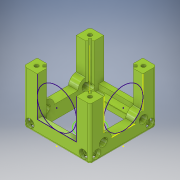
# Autodesk Inventor part: 10_Cube_v0_B
Saved by Autodesk Inventor 2019 (Build 230136000, 136)
## iProperties
Created: 2018-05-19
Part Number: 10_Cube_v0_B
Material: Generisch
Document SubType Name: Modeling
Designer: diederichbenedict
Density: 1 g/cm^3
Appearance: IPHT_Grün
Mass: 20.3218 g
Surface Area: 129.075 cm^2
Volume: 20.3218 cm^3
Author: diederichbenedict
Autodesk Inventor part; units mm, degrees
ref_plane "YZ Plane" through (0, 0, 0) normal (1, 0, 0) x (0, 1, 0)
ref_plane "XZ Plane" through (0, 0, 0) normal (0, 1, 0) x (-1, 0, 0)
sketch "Skizze1" plane through (0, 0, 0) normal (0, 0, 1) x (1, 0, 0)
  line L0 (-24.9, 24.9) -> (24.9, 24.9)
  line L1 (24.9, 24.9) -> (24.9, -24.9)
  line L2 (24.9, -24.9) -> (-24.9, -24.9)
  line L3 (-24.9, -24.9) -> (-24.9, 24.9)
  line L4 (-24.9, 24.9) -> (24.9, -24.9) construction
  line L5 (24.9, 24.9) -> (-24.9, -24.9) construction
  line L6 (14.6269, -17.9) -> (-14.6269, -17.9)
  line L7 (-17.9, -14.6269) -> (-17.9, 14.6269)
  line L8 (-14.6269, 17.9) -> (14.6269, 17.9)
  line L9 (17.9, 14.6269) -> (17.9, -14.6269)
  line L10 (20.5, -20.5) -> (-20.5, 20.5) construction
  line L11 (-20.5, -20.5) -> (20.5, 20.5) construction
  line L12 (-14.6269, 17.9) -> (-17.9, 14.6269)
  line L13 (-14.6269, 17.9) -> (-9.9981, 17.9) construction
  line L14 (17.9, -14.6269) -> (14.6269, -17.9)
  line L15 (17.9, -14.6269) -> (22.5288, -14.6269) construction
  line L16 (-17.9, -14.6269) -> (-14.6269, -17.9)
  line L17 (14.6269, 17.9) -> (17.9, 14.6269)
  point P0 (0, 0)
  dimension "d0" = 49.8
  dimension "d1" = 49.8
  dimension "d2" = 41
  dimension "d3" = 41
  dimension "d4" = 135
  dimension "d5" = 23
  dimension "d6" = 135
  dimension "d7" = 23
  dimension "a1" = 23
  dimension "d9" = 23
  dimension "a2" = 7
  dimension "d42" = 7
  dimension "d43" = 7
  dimension "d44" = 7
  constraints: 36 end point, 4 horizontal, 4 midpoint, 4 parallel, 4 perpendicular, 2 equal length
  measures "d0" distance of L1.end L2.end
  measures "d1" distance of L0.end L1.end
  measures "d2" distance of L10.end L11.end
  measures "d3" distance of L11.start L10.end
  measures "d4" angle of L12 L13
  measures "d5" distance from line of point (0, 0) L12
  measures "d6" angle of L14 L15
  measures "d7" distance from line of point (0, 0) L14
  measures "a1" distance from line of point (0, 0) L17
  measures "d9" distance from line of L16 point (0, 0)
  measures "a2" distance between parallel lines of L8 L0
  measures "d42" distance between parallel lines of L3 L7
  measures "d43" distance between parallel lines of L2 L6
  measures "d44" distance between parallel lines of L1 L9
extrude "Extrusion1" add sketch "Skizze1" along normal blind 10.3
sketch "Skizze2" plane through (0, 0, 10.3) normal (0, 0, 1) x (1, 0, 0)
  line L0 (-17.9, 14.6269) -> (-14.6269, 17.9) construction
  line L1 (-14.6269, 17.9) -> (14.6269, 17.9) construction
  line L2 (14.6269, 17.9) -> (17.9, 14.6269) construction
  line L3 (17.9, 14.6269) -> (17.9, -14.6269) construction
  line L4 (17.9, -14.6269) -> (14.6269, -17.9) construction
  line L5 (14.6269, -17.9) -> (-14.6269, -17.9) construction
  line L6 (-14.6269, -17.9) -> (-17.9, -14.6269) construction
  line L7 (-17.9, -14.6269) -> (-17.9, 14.6269) construction
  line L8 (24.9, 24.9) -> (-24.9, 24.9) construction
  line L9 (-24.9, 24.9) -> (-24.9, -24.9) construction
  line L10 (-24.9, -24.9) -> (24.9, -24.9) construction
  line L11 (24.9, -24.9) -> (24.9, 24.9) construction
  line L12 (-17.9, -14.6269) -> (-24.9, -14.6269)
  line L13 (-24.9, -24.9) -> (-24.9, 24.9) projected
  line L14 (-24.9, -14.6269) -> (-24.9, -24.9)
  line L15 (-17.9, -14.6269) -> (-14.6269, -17.9) projected
  line L16 (-17.9, -14.6269) -> (-14.6269, -17.9)
  line L17 (-14.6269, -17.9) -> (-14.6269, -24.9)
  line L18 (24.9, -24.9) -> (-24.9, -24.9) projected
  line L19 (-24.9, -24.9) -> (-14.6269, -24.9)
  line L20 (-17.9, -14.9) -> (-17.9, 14.9) projected
  line L21 (14.9, -17.9) -> (-14.9, -17.9) projected
  line L22 (17.9, 14.9) -> (17.9, -14.9) projected
  line L23 (-14.9, 17.9) -> (-9.9, 17.9) projected
  circle A0 centre (0, 0) radius 17.9
  line L24 (14.6269, -17.9) -> (17.9, -14.6269)
  line L25 (17.9, -14.6269) -> (24.9, -14.6269)
  line L26 (24.9, -24.9) -> (24.9, -14.6269)
  line L27 (14.6269, -24.9) -> (24.9, -24.9)
  line L28 (14.6269, -17.9) -> (14.6269, -24.9)
  line L29 (17.9, 14.6269) -> (14.6269, 17.9)
  line L30 (14.6269, 17.9) -> (14.6269, 24.9)
  line L31 (24.9, 24.9) -> (14.6269, 24.9)
  line L32 (24.9, 14.6269) -> (24.9, 24.9)
  line L33 (17.9, 14.6269) -> (24.9, 14.6269)
  line L34 (-14.6269, 17.9) -> (-17.9, 14.6269)
  line L35 (-17.9, 14.6269) -> (-24.9, 14.6269)
  line L36 (-24.9, 24.9) -> (-24.9, 14.6269)
  line L37 (-14.6269, 24.9) -> (-24.9, 24.9)
  line L38 (-14.6269, 17.9) -> (-14.6269, 24.9)
  line L39 (0, 0) -> (24.9, -24.9) construction
  line L40 (14.4957, -15.9099) -> (16.617, -18.0312)
  line L41 (16.617, -18.0312) -> (18.0312, -16.617)
  line L42 (18.0312, -16.617) -> (15.9099, -14.4957)
  line L43 (15.9099, -14.4957) -> (14.4957, -15.9099)
  line L44 (14.4957, -15.9099) -> (18.0312, -16.617) construction
  line L45 (16.617, -18.0312) -> (15.9099, -14.4957) construction
  line L46 (14.6269, -17.9) -> (17.9, -14.6269) projected
  point P0 (16.2635, -16.2635)
  point P1 (16.9706, -15.5563)
  point P2 (15.5563, -16.9706)
  dimension "d80" = 360
  dimension "d101" = 3
  dimension "d102" = 2
  constraints: 54 end point, 6 point on line, 5 midpoint, 3 perpendicular, 3 tangent, 2 collinear, 2 parallel, 1 centre point, 1 vertical, 41 other
  measures "d101" distance of L40.start L40.end
  measures "d102" distance of L41.end L40.end
extrude "Extrusion2" add sketch "Skizze2" along normal blind 29.4 contours L15 L17 L18 L13 L12 | L29 L30 L31 L32 L33 | L13 L37 L38 L34 L35 | L28 L24 L40 L41 L42 L25 L26 L18 | L24 L42 L41 L40
fillet "Rundung1" radius 2 8 edges at (24.9, 24.9, 19.85) (24.9, 0, 0) (24.9, -24.9, 19.85) (-24.9, 24.9, 19.85) (-24.9, -24.9, 19.85) (-24.9, 0, 0) (0, -24.9, 0) (0, 24.9, 0)
sketch "Skizze3" plane through (0, 0, 39.7) normal (0, 0, 1) x (1, 0, 0)
  line L0 (20, 20) -> (-20, 20) construction
  line L1 (-20, 20) -> (-20, -20) construction
  line L2 (-20, -20) -> (20, -20) construction
  line L3 (20, -20) -> (20, 20) construction
  line L4 (20, 20) -> (-20, -20) construction
  line L5 (-20, 20) -> (20, -20) construction
  line L6 (22.9, -22.9) -> (20.7681, -22.9) projected
  line L7 (22.9, -20.7681) -> (22.9, -22.9) projected
  arc A0 (20.7681, -22.9) -> (22.9, -20.7681) centre (20, -20) ccw projected
  point P0 (0, 0)
  point P1 (-20, 20)
  point P2 (20, -20)
  point P3 (20, -20)
  point P4 (20, -20)
  point P5 (-20, -20)
  point P6 (-20, -20)
  point P7 (-15.7881, 5.2)
  point P8 (-15.7881, -5.2)
  dimension "d15" = 40
  dimension "d16" = 40
  constraints: 12 end point, 2 midpoint, 2 parallel, 1 horizontal, 1 perpendicular
  measures "d15" distance of L2.end L1.end
  measures "d16" distance of L1.end L0.end
hole "Bohrung1" at (20, -20, 39.7) at (-20, -20, 39.7) at (-20, 20, 39.7) at (20, 20, 39.7) direction (0, 0, -1) diameter 2.9 depth 10 tip angle 118
sketch "Skizze4" plane through (0, 0, 0) normal (0, 0, -1) x (-1, 0, 0)
  circle A0 centre (20, -20) radius 1.45 projected
  circle A1 centre (20, 20) radius 1.45 projected
  line L0 (14.6269, 17.9) -> (17.9, 14.6269) projected
  line L1 (17.9, 14.6269) -> (17.9, -14.6269) projected
  line L2 (17.9, -14.6269) -> (14.6269, -17.9) projected
  line L3 (14.6269, -17.9) -> (-14.6269, -17.9) projected
  line L4 (-14.6269, -17.9) -> (-17.9, -14.6269) projected
  line L5 (-17.9, -14.6269) -> (-17.9, 14.6269) projected
  line L6 (-17.9, 14.6269) -> (-14.6269, 17.9) projected
  line L7 (-14.6269, 17.9) -> (14.6269, 17.9) projected
  line L8 (-22.9, 22.9) -> (22.9, 22.9) projected
  line L9 (-22.9, -22.9) -> (-22.9, 22.9) projected
  line L10 (22.9, -22.9) -> (-22.9, -22.9) projected
  line L11 (22.9, 22.9) -> (22.9, -22.9) projected
  circle A2 centre (-20, -20) radius 1.45 projected
  circle A3 centre (-20, 20) radius 1.45 projected
  point P0 (0, 0)
  point P1 (19.8136, -18.5116)
  point P2 (18.5116, -19.8136)
  point P3 (18.5116, 19.8136)
  point P4 (19.8136, 18.5116)
  point P5 (-18.5116, -19.8136)
  point P6 (-19.8136, -18.5116)
  point P7 (-19.8136, 18.5116)
  point P8 (-18.5116, 19.8136)
  constraints: 6 other
hole "Bohrung2" at (-20, -20, 0) at (-20, 20, 0) at (20, -20, 0) at (20, 20, 0) direction (0, 0, 1) diameter 3 depth 15 tip angle 118 counterbore diameter 6.2 counterbore depth 2.5
sketch "Skizze8" plane through (24.9, -14.6269, 10.3) normal (1, 0, 0) x (0, 0, -1)
  line L0 (-39.7, 33.8588) -> (-39.7, -4.605) projected
  arc A0 (-37.7, 39.5269) -> (-39.7, 37.5269) centre (-37.7, 37.5269) ccw projected
  arc A1 (8.3, -10.2731) -> (10.3, -8.2731) centre (8.3, -8.2731) ccw projected
  arc A2 (-39.7, -8.2731) -> (-37.7, -10.2731) centre (-37.7, -8.2731) ccw projected
  arc A3 (10.3, 37.5269) -> (8.3, 39.5269) centre (8.3, 37.5269) ccw projected
  line L1 (-37.7, -8.2731) -> (8.3, 37.5269) construction
  line L2 (8.3, -8.2731) -> (8.3, 37.5269) construction
  line L3 (8.3, -8.2731) -> (-37.7, 37.5269) construction
  circle A4 centre (-14.7, 14.6269) radius 6.587 construction
  line L4 (-34.7, -5.3731) -> (5.3, -5.3731) construction
  line L5 (5.3, -5.3731) -> (5.3, 34.6269) construction
  line L6 (5.3, 34.6269) -> (-34.7, 34.6269) construction
  line L7 (-34.7, 34.6269) -> (-34.7, -5.3731) construction
  line L8 (-34.7, -5.3731) -> (5.3, 34.6269) construction
  line L9 (5.3, -5.3731) -> (-34.7, 34.6269) construction
  point P0 (10.3, 14.6269)
  dimension "d110" = 40
  dimension "d111" = 40
  constraints: 16 end point, 3 midpoint, 2 parallel, 1 centre point, 1 horizontal, 1 perpendicular
  measures "d110" distance of L6.end L5.end
  measures "d111" distance of L5.end L4.end
sketch "Skizze9" plane through (14.6269, 17.9, 10.3) normal (-1, 0, 0) x (0, 0, 1)
  line L0 (-3.2288, -37.966) -> (32.6288, -37.966) construction
  line L1 (32.6288, -37.966) -> (34.766, -35.8288) construction
  line L2 (34.766, -35.8288) -> (34.766, 0.0288) construction
  line L3 (34.766, 0.0288) -> (32.6288, 2.166) construction
  line L4 (32.6288, 2.166) -> (-3.2288, 2.166) construction
  line L5 (-3.2288, 2.166) -> (-5.366, 0.0288) construction
  line L6 (-5.366, 0.0288) -> (-5.366, -35.8288) construction
  line L7 (-5.366, -35.8288) -> (-3.2288, -37.966) construction
  circle A0 centre (29.7, -2.9) radius 3.2639 construction
  circle A1 centre (-0.3, -2.9) radius 3.2639 construction
  circle A2 centre (-0.3, -32.9) radius 3.2639 construction
  circle A3 centre (29.7, -32.9) radius 3.2639 construction
  circle A4 centre (14.7, -17.9) radius 13.3985 construction
  line L8 (-3.643, 3.166) -> (33.043, 3.166)
  line L9 (33.043, 3.166) -> (35.766, 0.443)
  line L10 (35.766, 0.443) -> (35.766, -36.243)
  line L11 (35.766, -36.243) -> (33.043, -38.966)
  line L12 (33.043, -38.966) -> (-3.643, -38.966)
  line L13 (-3.643, -38.966) -> (-6.366, -36.243)
  line L14 (-6.366, -36.243) -> (-6.366, 0.443)
  line L15 (-6.366, 0.443) -> (-3.643, 3.166)
  point P0 (-10.3, -17.9)
  dimension "d82" = 1
  constraints: 16 end point, 7 other
  measures "d82" distance between parallel lines of L4 L8
extrude "Extrusion5" cut sketch "Skizze9" along normal up to surface (29.2538 mm away)
sketch "Skizze10" plane through (-24.9, -14.6269, 10.3) normal (-1, 0, 0) x (0, 0, 1)
  circle A0 centre (-0.3, 29.6269) radius 3.2639 construction
  circle A1 centre (-0.3, -0.3731) radius 3.2639 construction
  circle A2 centre (29.7, 29.6269) radius 3.2639 construction
  circle A3 centre (29.7, -0.3731) radius 3.2639 construction
  circle A4 centre (29.7, 29.6269) radius 3.3139
  circle A5 centre (29.7, -0.3731) radius 3.3139
  line L0 (-8.3, -10.2731) -> (29.4, -10.2731) projected
  line L1 (29.4, 39.5269) -> (-8.3, 39.5269) projected
  circle A6 centre (-0.3, -0.3731) radius 2.95
  circle A7 centre (-0.3, 29.6269) radius 2.95
  point P0 (-10.3, 14.6269)
  dimension "a4" = 0.05
  dimension "d90" = 0.05
  dimension "d130" = 9.9
  dimension "d131" = 9.9
  dimension "d132" = 5.9
  dimension "d133" = 5.9
  constraints: 4 centre point, 2 coincident
  measures "a4" radial gap between concentric circles of A2 A4
  measures "d90" radial gap between concentric circles of A3 A5
  measures "d130" distance from line of L0 A1.centre
  measures "d131" distance from line of L1 A0.centre
  measures "d132" diameter of A6
  measures "d133" diameter of A7
extrude "Extrusion6" cut sketch "Skizze10" against normal through all contours A6 | A7
sketch "Skizze11" plane through (-24.9, -22.9, 2) normal (-1, 0, 0) x (0, 0, 1)
  line L0 (10.9263, 37.5269) -> (37.7, 37.5269) construction
  line L1 (37.7, 45.8) -> (37.7, 37.5269) construction
  line L2 (0, 45.8) -> (37.7, 45.8) construction
  line L3 (0, 0) -> (0, 45.8) construction
  line L4 (37.7, 0) -> (0, 0) construction
  line L5 (37.7, 8.2731) -> (37.7, 0) construction
  line L6 (10.9263, 8.2731) -> (37.7, 8.2731) construction
  line L7 (8.3, 34.9653) -> (8.3, 10.8347) construction
  arc A0 (8.3, 34.7503) -> (11.1419, 37.5269) centre (8.1696, 37.7265) ccw
  line L8 (10.9263, 8.2731) -> (37.7, 8.2731) projected
  line L9 (8.3, 10.8347) -> (8.3, 34.7503) projected
  arc A1 (11.1419, 8.2731) -> (8.3, 11.0497) centre (8.1696, 8.0735) ccw
  line L10 (8.1696, 8.0735) -> (14.1696, 8.0735) construction
  line L11 (14.1696, 8.0735) -> (14.1696, 14.0735) construction
  line L12 (14.1696, 14.0735) -> (8.1696, 14.0735) construction
  line L13 (8.1696, 14.0735) -> (8.1696, 8.0735) construction
  line L14 (8.1696, 37.7265) -> (14.1696, 37.7265) construction
  line L15 (14.1696, 37.7265) -> (14.1696, 31.7265) construction
  line L16 (14.1696, 31.7265) -> (8.1696, 31.7265) construction
  line L17 (8.1696, 31.7265) -> (8.1696, 37.7265) construction
  arc A2 (8.3, 31.7265) -> (14.1696, 37.5269) centre (8, 37.9) ccw
  arc A3 (14.1696, 8.2731) -> (8.3, 14.0735) centre (8, 7.9) ccw
  line L18 (11.1419, 37.5269) -> (37.7, 37.5269) projected
  line L19 (14.1696, 37.5269) -> (11.1419, 37.5269)
  line L20 (8.3, 34.7503) -> (8.3, 31.7265)
  line L21 (8.3, 14.0735) -> (8.3, 11.0497)
  line L22 (11.1419, 8.2731) -> (14.1696, 8.2731)
  arc A4 (8.3, 10.8347) -> (10.9263, 8.2731) centre (8, 7.9) ccw projected
  arc A5 (10.9263, 37.5269) -> (8.3, 34.9653) centre (8, 37.9) ccw projected
  dimension "d124" = 6
  dimension "d125" = 6
  dimension "d126" = 6
  dimension "d127" = 6
  constraints: 24 end point, 8 point on circle, 8 point on line, 5 parallel, 4 centre point, 3 perpendicular, 2 collinear, 2 horizontal
  measures "d124" distance of L12.end L11.end
  measures "d125" distance of L11.end L10.end
  measures "d126" distance of L15.end L16.end
  measures "d127" distance of L14.end L15.end
extrude "Extrusion7" add sketch "Skizze11" against normal up to surface (7 mm away) contours A3 L8 A1 L9 | A0 L18 A2 L9
sketch "Skizze12" plane through (24.9, -22.9, 2) normal (1, 0, 0) x (0, 0, -1)
  arc A0 (-8.3, 14.0735) -> (-14.1696, 8.2731) centre (-8, 7.9) ccw projected
  arc A1 (-14.1696, 37.5269) -> (-8.3, 31.7265) centre (-8, 37.9) ccw projected
  arc A2 (-11.1419, 37.5269) -> (-8.3, 34.7503) centre (-8.1696, 37.7265) ccw projected
  arc A3 (-8.3, 11.0497) -> (-11.1419, 8.2731) centre (-8.1696, 8.0735) ccw projected
  line L0 (-8.3, 8.2731) -> (-37.7, 8.2731) projected
  line L1 (-14.1696, 8.2731) -> (-11.1419, 8.2731)
  line L2 (-8.3, 11.0497) -> (-8.3, 14.0735)
  line L3 (-8.3, 37.5269) -> (-8.3, 8.2731) projected
  line L4 (-8.3, 34.7503) -> (-8.3, 31.7265)
  line L5 (-14.1696, 37.5269) -> (-11.1419, 37.5269)
  constraints: 8 end point, 2 collinear, 1 perpendicular, 1 vertical
ref_plane "Arbeitsebene1" through (17.9, -21.066, 43) normal (-1, 0, 0) x (0, 0, 1)
extrude "Extrusion8" add sketch "Skizze12" against normal up to surface (7 mm away) contours L2 A3 L0 A0 | A1 L5 A2 L3
sketch "Skizze13" plane through (0, 0, 39.7) normal (0, 0, 1) x (1, 0, 0)
  arc A0 (22.9, -24.9) -> (24.9, -22.9) centre (22.9, -22.9) ccw construction
  line L0 (17.9, -14.6269) -> (14.6269, -17.9) construction
  line L1 (14.6269, -17.9) -> (14.6269, -24.9) construction
  line L2 (14.6269, -24.9) -> (22.9, -24.9) construction
  line L3 (16.9706, -18.3848) -> (-18.3848, 16.9706)
  line L4 (-18.3848, 16.9706) -> (-16.9706, 18.3848)
  line L5 (-16.9706, 18.3848) -> (18.3848, -16.9706)
  line L6 (18.3848, -16.9706) -> (16.9706, -18.3848)
  line L7 (16.9706, -18.3848) -> (-16.9706, 18.3848) construction
  line L8 (-18.3848, 16.9706) -> (18.3848, -16.9706) construction
  line L9 (16.9706, -18.3848) -> (66.9706, -18.3848) construction
  line L10 (18.3848, 16.9706) -> (-16.9706, -18.3848)
  line L11 (-16.9706, -18.3848) -> (-18.3848, -16.9706)
  line L12 (-18.3848, -16.9706) -> (16.9706, 18.3848)
  line L13 (16.9706, 18.3848) -> (18.3848, 16.9706)
  line L14 (18.3848, 16.9706) -> (-18.3848, -16.9706) construction
  line L15 (-16.9706, -18.3848) -> (16.9706, 18.3848) construction
  line L16 (24.9, -22.9) -> (24.9, -14.6269) projected
  line L17 (24.9, -14.6269) -> (17.9, -14.6269) projected
  line L18 (22.9, -22.9) -> (20.7681, -22.9) projected
  line L19 (22.9, -20.7681) -> (22.9, -22.9) projected
  arc A1 (20.7681, -22.9) -> (22.9, -20.7681) centre (20, -20) ccw projected
  point P0 (0, 0)
  point P1 (20, -20)
  point P2 (20, -20)
  point P3 (-20, -20)
  point P4 (20, -20)
  point P5 (-20, -20)
  point P6 (-20, -20)
  point P7 (-20, -20)
  point P8 (-15.7881, 5.2)
  point P9 (-15.7881, -5.2)
  dimension "d103" = 50
  dimension "d104" = 135
  dimension "d105" = 2
  dimension "d106" = 50
  dimension "d107" = 2
  constraints: 26 end point, 5 parallel, 4 midpoint, 2 perpendicular, 1 equal length, 1 horizontal
  measures "d103" distance of L3.start L3.end
  measures "d104" angle of L9 L3
  measures "d105" distance of L3.end L4.end
  measures "d106" distance of L10.start L10.end
  measures "d107" distance of L10.end L11.end
extrude "Extrusion9" cut sketch "Skizze13" against normal up to surface (29.4 mm away) contours L3 L10 L5 L6 | L10 L11 L12 L3 | L3 L12 L5 L10 | L3 L4 L5 L12 | L5 L12 L13 L10
hole "Bohrung3" at (24.9, -20, 5) at (24.9, 20, 5) at (24.9, -20, 45) at (24.9, 20, 45) direction (-1, 0, 0) diameter 3 depth 15 tip angle 118 counterbore diameter 6.2 counterbore depth 2.5
sketch "Skizze14" plane through (0, 0, 0) normal (0, 0, -1) x (-1, 0, 0)
  circle A0 centre (0, 0) radius 9.428
  constraints: 1 centre point, 1 coincident
pattern_circular "Runde Anordnung2" count 4 over 360 about axis through (0, 0, 0) along (0, 0, 1) of "Bohrung3"
sketch "Sketch15" plane through (24.9, 14.6269, 39.7) normal (1, 0, 0) x (0, 0, -1)
  line L0 (23.5304, 0) -> (0, 0) projected
  line L1 (29.4, -23.4534) -> (29.4, -5.8005) projected
  line L2 (23.5304, -29.2538) -> (0, -29.2538) projected
  circle A0 centre (14.7731, -14.6269) radius 14.6269
  point P0 (39.7, -14.6269)
  constraints: 3 tangent, 1 centre point
sketch "Sketch16" plane through (-14.6269, -24.9, 10.3) normal (0, -1, 0) x (1, 0, 0)
  line L0 (29.2538, 0) -> (29.2538, 29.4)
  line L1 (29.2538, 0) -> (0, 0)
  line L2 (0, 0) -> (0, 29.4)
  circle A0 centre (14.6269, 14.6269) radius 14.6269
  point P0 (14.6269, -10.3)
  constraints: 6 end point, 3 tangent, 2 vertical, 1 centre point, 1 horizontal, 4 other
sketch "Sketch17" plane through (-14.6269, 24.9, 10.3) normal (0, 1, 0) x (1, 0, 0)
  arc A0 (33.8459, 8.3) -> (37.5269, 4.2046) centre (34.6269, 5.3) ccw projected
  line L0 (-4.5921, 8.3) -> (33.8459, 8.3) projected
  arc A1 (-8.2731, 4.2046) -> (-4.5921, 8.3) centre (-5.3731, 5.3) ccw projected
  line L1 (-8.2731, -29.4) -> (-8.2731, 4.2046) projected
  line L2 (0, -29.4) -> (-8.2731, -29.4) projected
  line L3 (0, 0) -> (0, -29.4) projected
  line L4 (29.2538, 0) -> (0, 0) projected
  line L5 (29.2538, 0) -> (29.2538, -29.4) projected
  line L6 (37.5269, -29.4) -> (29.2538, -29.4) projected
  line L7 (37.5269, 4.2046) -> (37.5269, -29.4) projected
  line L8 (29.2538, 2) -> (-40.4916, 2) construction
  line L9 (-40.4916, 2) -> (-40.4916, 5.7242) construction
  line L10 (-40.4916, 5.7242) -> (29.2538, 5.7242) construction
  line L11 (29.2538, 5.7242) -> (29.2538, 2) construction
  line L12 (29.2538, 0) -> (29.2538, -29.4) projected
  spline S0 degree 2 poles (27.9167, 4.6013) (28.4799, 4.6013) (29.1404, 3.9206) (29.1404, 3.3047) knots 0 0 0 1 2 2 2
  spline S1 degree 2 poles (29.1404, 3.3047) (29.1404, 2.7111) (28.4779, 2.0041) (27.9147, 2.0041) knots 0 0 0 1 2 2 2
  spline S2 degree 2 poles (27.9147, 2.0041) (27.7668, 2.0041) (27.5277, 2.0385) (27.4183, 2.0669) knots 0 0 0 1 2 2 2
  spline S3 degree 2 poles (27.4183, 2.0669) (27.3332, 2.0932) (27.1327, 2.1803) (27.0699, 2.2127) knots 0 0 0 1 2 2 2
  line L13 (27.0699, 2.2127) -> (27.0699, 2.8083)
  line L14 (27.0699, 2.8083) -> (27.1327, 2.8083)
  spline S4 degree 2 poles (27.1327, 2.8083) (27.1793, 2.7678) (27.317, 2.6544) (27.4041, 2.6017) knots 0 0 0 1 2 2 2
  spline S5 degree 2 poles (27.4041, 2.6017) (27.4913, 2.547) (27.6999, 2.472) (27.8154, 2.472) knots 0 0 0 1 2 2 2
  spline S6 degree 2 poles (27.8154, 2.472) (27.9511, 2.472) (28.176, 2.5571) (28.2794, 2.6645) knots 0 0 0 1 2 2 2
  spline S7 degree 2 poles (28.2794, 2.6645) (28.3725, 2.7597) (28.4921, 3.0859) (28.4921, 3.3067) knots 0 0 0 1 2 2 2
  spline S8 degree 2 poles (28.4921, 3.3067) (28.4921, 3.5397) (28.3685, 3.8578) (28.2672, 3.955) knots 0 0 0 1 2 2 2
  spline S9 degree 2 poles (28.2672, 3.955) (28.17, 4.0502) (27.9309, 4.1333) (27.8114, 4.1333) knots 0 0 0 1 2 2 2
  spline S10 degree 2 poles (27.8114, 4.1333) (27.6878, 4.1333) (27.4629, 4.0502) (27.3859, 3.9996) knots 0 0 0 1 2 2 2
  spline S11 degree 2 poles (27.3859, 3.9996) (27.3008, 3.9489) (27.1732, 3.8416) (27.1266, 3.799) knots 0 0 0 1 2 2 2
  line L15 (27.1266, 3.799) -> (27.0699, 3.799)
  line L16 (27.0699, 3.799) -> (27.0699, 4.3865)
  spline S12 degree 2 poles (27.0699, 4.3865) (27.1388, 4.419) (27.3191, 4.5) (27.4163, 4.5284) knots 0 0 0 1 2 2 2
  spline S13 degree 2 poles (27.4163, 4.5284) (27.5338, 4.5648) (27.7384, 4.6013) (27.9167, 4.6013) knots 0 0 0 1 2 2 2
  spline S14 degree 2 poles (24.424, 3.3027) (24.424, 3.9105) (25.0723, 4.6053) (25.6355, 4.6053) knots 0 0 0 1 2 2 2
  spline S15 degree 2 poles (25.6355, 4.6053) (26.2007, 4.6053) (26.845, 3.9023) (26.845, 3.3027) knots 0 0 0 1 2 2 2
  spline S16 degree 2 poles (26.845, 3.3027) (26.845, 2.701) (26.2007, 2) (25.6355, 2) knots 0 0 0 1 2 2 2
  spline S17 degree 2 poles (25.6355, 2) (25.0723, 2) (24.424, 2.6969) (24.424, 3.3027) knots 0 0 0 1 2 2 2
  spline S18 degree 2 poles (25.0723, 3.3027) (25.0723, 3.0778) (25.1635, 2.7638) (25.2425, 2.6645) knots 0 0 0 1 2 2 2
  spline S19 degree 2 poles (25.2425, 2.6645) (25.3215, 2.5612) (25.5241, 2.472) (25.6335, 2.472) knots 0 0 0 1 2 2 2
  spline S20 degree 2 poles (25.6335, 2.472) (25.749, 2.472) (25.9374, 2.5551) (26.0245, 2.6605) knots 0 0 0 1 2 2 2
  spline S21 degree 2 poles (26.0245, 2.6605) (26.1015, 2.7577) (26.1967, 3.0798) (26.1967, 3.3027) knots 0 0 0 1 2 2 2
  spline S22 degree 2 poles (26.1967, 3.3027) (26.1967, 3.5336) (26.1055, 3.8375) (26.0265, 3.9408) knots 0 0 0 1 2 2 2
  spline S23 degree 2 poles (26.0265, 3.9408) (25.9475, 4.0442) (25.7429, 4.1333) (25.6335, 4.1333) knots 0 0 0 1 2 2 2
  spline S24 degree 2 poles (25.6335, 4.1333) (25.5221, 4.1333) (25.3154, 4.0381) (25.2405, 3.9368) knots 0 0 0 1 2 2 2
  spline S25 degree 2 poles (25.2405, 3.9368) (25.1594, 3.8274) (25.0723, 3.5377) (25.0723, 3.3027) knots 0 0 0 1 2 2 2
  line L17 (21.9098, 4.5527) -> (22.5135, 4.5527)
  line L18 (22.5135, 4.5527) -> (23.4779, 2.8104)
  line L19 (23.4779, 2.8104) -> (23.4779, 4.5527)
  line L20 (23.4779, 4.5527) -> (24.0512, 4.5527)
  line L21 (24.0512, 4.5527) -> (24.0512, 2.0527)
  line L22 (24.0512, 2.0527) -> (23.2814, 2.0527)
  line L23 (23.2814, 2.0527) -> (22.4832, 3.485)
  line L24 (22.4832, 3.485) -> (22.4832, 2.0527)
  line L25 (22.4832, 2.0527) -> (21.9098, 2.0527)
  line L26 (21.9098, 2.0527) -> (21.9098, 4.5527)
  spline S26 degree 2 poles (20.3235, 4.6013) (20.8867, 4.6013) (21.5472, 3.9206) (21.5472, 3.3047) knots 0 0 0 1 2 2 2
  spline S27 degree 2 poles (21.5472, 3.3047) (21.5472, 2.7111) (20.8847, 2.0041) (20.3215, 2.0041) knots 0 0 0 1 2 2 2
  spline S28 degree 2 poles (20.3215, 2.0041) (20.1736, 2.0041) (19.9345, 2.0385) (19.8251, 2.0669) knots 0 0 0 1 2 2 2
  spline S29 degree 2 poles (19.8251, 2.0669) (19.74, 2.0932) (19.5395, 2.1803) (19.4767, 2.2127) knots 0 0 0 1 2 2 2
  line L27 (19.4767, 2.2127) -> (19.4767, 2.8083)
  line L28 (19.4767, 2.8083) -> (19.5395, 2.8083)
  spline S30 degree 2 poles (19.5395, 2.8083) (19.5861, 2.7678) (19.7238, 2.6544) (19.811, 2.6017) knots 0 0 0 1 2 2 2
  spline S31 degree 2 poles (19.811, 2.6017) (19.8981, 2.547) (20.1067, 2.472) (20.2222, 2.472) knots 0 0 0 1 2 2 2
  spline S32 degree 2 poles (20.2222, 2.472) (20.358, 2.472) (20.5828, 2.5571) (20.6862, 2.6645) knots 0 0 0 1 2 2 2
  spline S33 degree 2 poles (20.6862, 2.6645) (20.7794, 2.7597) (20.8989, 3.0859) (20.8989, 3.3067) knots 0 0 0 1 2 2 2
  spline S34 degree 2 poles (20.8989, 3.3067) (20.8989, 3.5397) (20.7753, 3.8578) (20.674, 3.955) knots 0 0 0 1 2 2 2
  spline S35 degree 2 poles (20.674, 3.955) (20.5768, 4.0502) (20.3377, 4.1333) (20.2182, 4.1333) knots 0 0 0 1 2 2 2
  spline S36 degree 2 poles (20.2182, 4.1333) (20.0946, 4.1333) (19.8697, 4.0502) (19.7927, 3.9996) knots 0 0 0 1 2 2 2
  spline S37 degree 2 poles (19.7927, 3.9996) (19.7076, 3.9489) (19.58, 3.8416) (19.5334, 3.799) knots 0 0 0 1 2 2 2
  line L29 (19.5334, 3.799) -> (19.4767, 3.799)
  line L30 (19.4767, 3.799) -> (19.4767, 4.3865)
  spline S38 degree 2 poles (19.4767, 4.3865) (19.5456, 4.419) (19.7259, 4.5) (19.8231, 4.5284) knots 0 0 0 1 2 2 2
  spline S39 degree 2 poles (19.8231, 4.5284) (19.9406, 4.5648) (20.1452, 4.6013) (20.3235, 4.6013) knots 0 0 0 1 2 2 2
  line L31 (19.3754, 4.5527) -> (18.5306, 2.0527)
  line L32 (18.5306, 2.0527) -> (17.8458, 2.0527)
  line L33 (17.8458, 2.0527) -> (17.001, 4.5527)
  line L34 (17.001, 4.5527) -> (17.6473, 4.5527)
  line L35 (17.6473, 4.5527) -> (17.8033, 4.0421)
  line L36 (17.8033, 4.0421) -> (18.5893, 4.0421)
  line L37 (18.5893, 4.0421) -> (18.7473, 4.5527)
  line L38 (18.7473, 4.5527) -> (19.3754, 4.5527)
  line L39 (17.941, 3.5883) -> (18.1963, 2.7618)
  line L40 (18.1963, 2.7618) -> (18.4536, 3.5883)
  line L41 (18.4536, 3.5883) -> (17.941, 3.5883)
  line L42 (14.6651, 2.0527) -> (15.5241, 4.5527)
  line L43 (15.5241, 4.5527) -> (16.1785, 4.5527)
  line L44 (16.1785, 4.5527) -> (17.0375, 2.0527)
  line L45 (17.0375, 2.0527) -> (16.3871, 2.0527)
  line L46 (16.3871, 2.0527) -> (15.8422, 3.7484)
  line L47 (15.8422, 3.7484) -> (15.2992, 2.0527)
  line L48 (15.2992, 2.0527) -> (14.6651, 2.0527)
  line L49 (14.4321, 4.5527) -> (14.4321, 2.0527)
  line L50 (14.4321, 2.0527) -> (12.7425, 2.0527)
  line L51 (12.7425, 2.0527) -> (12.7425, 2.5288)
  line L52 (12.7425, 2.5288) -> (13.8081, 2.5288)
  line L53 (13.8081, 2.5288) -> (13.8081, 2.9684)
  line L54 (13.8081, 2.9684) -> (12.8255, 2.9684)
  line L55 (12.8255, 2.9684) -> (12.8255, 3.4445)
  line L56 (12.8255, 3.4445) -> (13.8081, 3.4445)
  line L57 (13.8081, 3.4445) -> (13.8081, 4.0766)
  line L58 (13.8081, 4.0766) -> (12.7425, 4.0766)
  line L59 (12.7425, 4.0766) -> (12.7425, 4.5527)
  line L60 (12.7425, 4.5527) -> (14.4321, 4.5527)
  line L61 (10.2729, 3.6815) -> (11.3851, 3.6815)
  line L62 (11.3851, 3.6815) -> (11.3851, 3.2156)
  line L63 (11.3851, 3.2156) -> (10.2729, 3.2156)
  line L64 (10.2729, 3.2156) -> (10.2729, 3.6815)
  spline S40 degree 2 poles (8.0524, 3.7058) (8.0524, 3.9023) (8.1862, 4.2346) (8.3178, 4.3541) knots 0 0 0 1 2 2 2
  spline S41 degree 2 poles (8.3178, 4.3541) (8.4495, 4.4737) (8.8101, 4.6053) (9.0735, 4.6053) knots 0 0 0 1 2 2 2
  spline S42 degree 2 poles (9.0735, 4.6053) (9.3531, 4.6033) (9.7542, 4.5122) (9.8859, 4.4534) knots 0 0 0 1 2 2 2
  line L65 (9.8859, 4.4534) -> (9.8859, 3.9084)
  line L66 (9.8859, 3.9084) -> (9.8292, 3.9084)
  spline S43 degree 2 poles (9.8292, 3.9084) (9.7806, 3.9348) (9.6631, 4.0036) (9.5678, 4.0401) knots 0 0 0 1 2 2 2
  spline S44 degree 2 poles (9.5678, 4.0401) (9.4787, 4.0746) (9.2943, 4.1212) (9.1829, 4.1212) knots 0 0 0 1 2 2 2
  spline S45 degree 2 poles (9.1829, 4.1212) (9.0857, 4.1212) (8.8588, 4.0725) (8.7899, 4.0077) knots 0 0 0 1 2 2 2
  spline S46 degree 2 poles (8.7899, 4.0077) (8.7392, 3.9571) (8.6825, 3.8335) (8.6825, 3.7301) knots 0 0 0 1 2 2 2
  spline S47 degree 2 poles (8.6825, 3.7301) (8.6825, 3.641) (8.7554, 3.5154) (8.8142, 3.4769) knots 0 0 0 1 2 2 2
  spline S48 degree 2 poles (8.8142, 3.4769) (8.8993, 3.4202) (9.1424, 3.3878) (9.2295, 3.3878) knots 0 0 0 1 2 2 2
  spline S49 degree 2 poles (9.2295, 3.3878) (9.3673, 3.3878) (9.6286, 3.4323) (9.7238, 3.4566) knots 0 0 0 1 2 2 2
  line L67 (9.7238, 3.4566) -> (9.7785, 3.4566)
  line L68 (9.7785, 3.4566) -> (9.7785, 2.0527)
  line L69 (9.7785, 2.0527) -> (8.1213, 2.0527)
  line L70 (8.1213, 2.0527) -> (8.1213, 2.5247)
  line L71 (8.1213, 2.5247) -> (9.1849, 2.5247)
  line L72 (9.1849, 2.5247) -> (9.1849, 2.94)
  spline S50 degree 2 poles (9.1849, 2.94) (9.1343, 2.936) (8.9945, 2.9319) (8.956, 2.9319) knots 0 0 0 1 2 2 2
  spline S51 degree 2 poles (8.956, 2.9319) (8.7757, 2.9319) (8.4718, 3.0049) (8.3523, 3.0798) knots 0 0 0 1 2 2 2
  spline S52 degree 2 poles (8.3523, 3.0798) (8.2105, 3.173) (8.0524, 3.483) (8.0524, 3.7058) knots 0 0 0 1 2 2 2
  spline S53 degree 2 poles (5.8381, 3.3027) (5.8381, 3.6268) (5.9414, 4.113) (6.0569, 4.2771) knots 0 0 0 1 2 2 2
  spline S54 degree 2 poles (6.0569, 4.2771) (6.1704, 4.4392) (6.537, 4.6053) (6.8004, 4.6053) knots 0 0 0 1 2 2 2
  spline S55 degree 2 poles (6.8004, 4.6053) (7.0658, 4.6053) (7.4305, 4.4392) (7.546, 4.2731) knots 0 0 0 1 2 2 2
  spline S56 degree 2 poles (7.546, 4.2731) (7.6614, 4.109) (7.7648, 3.6268) (7.7648, 3.3027) knots 0 0 0 1 2 2 2
  spline S57 degree 2 poles (7.7648, 3.3027) (7.7648, 2.9704) (7.6614, 2.5004) (7.5439, 2.3302) knots 0 0 0 1 2 2 2
  spline S58 degree 2 poles (7.5439, 2.3302) (7.4264, 2.1641) (7.0557, 2.002) (6.8004, 2.002) knots 0 0 0 1 2 2 2
  spline S59 degree 2 poles (6.8004, 2.002) (6.531, 2.002) (6.1704, 2.1722) (6.0549, 2.3404) knots 0 0 0 1 2 2 2
  spline S60 degree 2 poles (6.0549, 2.3404) (5.9414, 2.5045) (5.8381, 2.9887) (5.8381, 3.3027) knots 0 0 0 1 2 2 2
  spline S61 degree 2 poles (6.4682, 3.3027) (6.4682, 2.8387) (6.6201, 2.4639) (6.8004, 2.4639) knots 0 0 0 1 2 2 2
  spline S62 degree 2 poles (6.8004, 2.4639) (6.9807, 2.4639) (7.1347, 2.8387) (7.1347, 3.3047) knots 0 0 0 1 2 2 2
  spline S63 degree 2 poles (7.1347, 3.3047) (7.1347, 3.7626) (6.9807, 4.1434) (6.8004, 4.1434) knots 0 0 0 1 2 2 2
  spline S64 degree 2 poles (6.8004, 4.1434) (6.6221, 4.1434) (6.4682, 3.7626) (6.4682, 3.3027) knots 0 0 0 1 2 2 2
  line L73 (3.2307, 4.5527) -> (3.2307, 3.6106)
  spline S65 degree 2 poles (3.2307, 3.6106) (3.2307, 3.4708) (3.2409, 3.2804) (3.2652, 3.2196) knots 0 0 0 1 2 2 2
  spline S66 degree 2 poles (3.2652, 3.2196) (3.2915, 3.1588) (3.3969, 3.1041) (3.4921, 3.1041) knots 0 0 0 1 2 2 2
  spline S67 degree 2 poles (3.4921, 3.1041) (3.5589, 3.1041) (3.6886, 3.1629) (3.7656, 3.2176) knots 0 0 0 1 2 2 2
  line L74 (3.7656, 3.2176) -> (3.7656, 4.5527)
  line L75 (3.7656, 4.5527) -> (4.3571, 4.5527)
  line L76 (4.3571, 4.5527) -> (4.3571, 3.6106)
  spline S68 degree 2 poles (4.3571, 3.6106) (4.3571, 3.4729) (4.3693, 3.2804) (4.3936, 3.2196) knots 0 0 0 1 2 2 2
  spline S69 degree 2 poles (4.3936, 3.2196) (4.42, 3.1588) (4.5253, 3.1041) (4.6205, 3.1041) knots 0 0 0 1 2 2 2
  spline S70 degree 2 poles (4.6205, 3.1041) (4.6914, 3.1041) (4.8312, 3.171) (4.896, 3.2176) knots 0 0 0 1 2 2 2
  line L77 (4.896, 3.2176) -> (4.896, 4.5527)
  line L78 (4.896, 4.5527) -> (5.4836, 4.5527)
  line L79 (5.4836, 4.5527) -> (5.4836, 2.6665)
  line L80 (5.4836, 2.6665) -> (4.896, 2.6665)
  line L81 (4.896, 2.6665) -> (4.896, 2.8752)
  spline S71 degree 2 poles (4.896, 2.8752) (4.7522, 2.7536) (4.4949, 2.6159) (4.3349, 2.6159) knots 0 0 0 1 2 2 2
  spline S72 degree 2 poles (4.3349, 2.6159) (4.1627, 2.6159) (3.8993, 2.78) (3.8304, 2.9441) knots 0 0 0 1 2 2 2
  spline S73 degree 2 poles (3.8304, 2.9441) (3.6623, 2.7861) (3.3624, 2.6159) (3.2084, 2.6159) knots 0 0 0 1 2 2 2
  spline S74 degree 2 poles (3.2084, 2.6159) (3.0768, 2.6159) (2.8681, 2.6989) (2.7972, 2.784) knots 0 0 0 1 2 2 2
  spline S75 degree 2 poles (2.7972, 2.784) (2.7182, 2.8752) (2.6392, 3.1244) (2.6392, 3.325) knots 0 0 0 1 2 2 2
  line L82 (2.6392, 3.325) -> (2.6392, 4.5527)
  line L83 (2.6392, 4.5527) -> (3.2307, 4.5527)
  line L84 (-0.0472, 4.5527) -> (-0.0472, 3.6106)
  spline S76 degree 2 poles (-0.0472, 3.6106) (-0.0472, 3.4708) (-0.0371, 3.2804) (-0.0128, 3.2196) knots 0 0 0 1 2 2 2
  spline S77 degree 2 poles (-0.0128, 3.2196) (0.0135, 3.1588) (0.1189, 3.1041) (0.2141, 3.1041) knots 0 0 0 1 2 2 2
  spline S78 degree 2 poles (0.2141, 3.1041) (0.281, 3.1041) (0.4106, 3.1629) (0.4876, 3.2176) knots 0 0 0 1 2 2 2
  line L85 (0.4876, 3.2176) -> (0.4876, 4.5527)
  line L86 (0.4876, 4.5527) -> (1.0792, 4.5527)
  line L87 (1.0792, 4.5527) -> (1.0792, 3.6106)
  spline S79 degree 2 poles (1.0792, 3.6106) (1.0792, 3.4729) (1.0913, 3.2804) (1.1157, 3.2196) knots 0 0 0 1 2 2 2
  spline S80 degree 2 poles (1.1157, 3.2196) (1.142, 3.1588) (1.2473, 3.1041) (1.3426, 3.1041) knots 0 0 0 1 2 2 2
  spline S81 degree 2 poles (1.3426, 3.1041) (1.4135, 3.1041) (1.5533, 3.171) (1.6181, 3.2176) knots 0 0 0 1 2 2 2
  line L88 (1.6181, 3.2176) -> (1.6181, 4.5527)
  line L89 (1.6181, 4.5527) -> (2.2056, 4.5527)
  line L90 (2.2056, 4.5527) -> (2.2056, 2.6665)
  line L91 (2.2056, 2.6665) -> (1.6181, 2.6665)
  line L92 (1.6181, 2.6665) -> (1.6181, 2.8752)
  spline S82 degree 2 poles (1.6181, 2.8752) (1.4742, 2.7536) (1.217, 2.6159) (1.0569, 2.6159) knots 0 0 0 1 2 2 2
  spline S83 degree 2 poles (1.0569, 2.6159) (0.8847, 2.6159) (0.6213, 2.78) (0.5524, 2.9441) knots 0 0 0 1 2 2 2
  spline S84 degree 2 poles (0.5524, 2.9441) (0.3843, 2.7861) (0.0845, 2.6159) (-0.0695, 2.6159) knots 0 0 0 1 2 2 2
  spline S85 degree 2 poles (-0.0695, 2.6159) (-0.2012, 2.6159) (-0.4099, 2.6989) (-0.4808, 2.784) knots 0 0 0 1 2 2 2
  spline S86 degree 2 poles (-0.4808, 2.784) (-0.5598, 2.8752) (-0.6388, 3.1244) (-0.6388, 3.325) knots 0 0 0 1 2 2 2
  line L93 (-0.6388, 3.325) -> (-0.6388, 4.5527)
  line L94 (-0.6388, 4.5527) -> (-0.0472, 4.5527)
  point P0 (14.6269, 10.3)
  dimension "d134" = 2
  constraints: 1 collinear, 2 other
  measures "d134" distance between parallel lines of L4 L8
extrude "Extrusion10" cut sketch "Sketch17" against normal blind 1 contours S0 S1 S2 S3 L13 L14 S4 S5 S6 S7 S8 S9 S10 S11 L15 L16 S12 S13 | S14 S15 S16 S17 | L17 L18 L19 L20 L21 L22 L23 L24 L25 L26 | S26 S27 S28 S29 L27 L28 S30 S31 S32 S33 S34 S35 S36 S37 L29 L30 S38 S39 | L31 L32 L33 L34 L35 L36 L37 L38 | L42 L43 L44 L45 L46 L47 L48 | L49 L50 L51 L52 L53 L54 L55 L56 L57 L58 L59 L60 | L61 L62 L63 L64 | S40 S41 S42 L65 L66 S43 S44 S45 S46 S47 S48 S49 L67 L68 L69 L70 L71 L72 S50 S51 S52 | S53 S54 S55 S56 S57 S58 S59 S60 | L73 S65 S66 S67 L74 L75 L76 S68 S69 S70 L77 L78 L79 L80 L81 S71 S72 S73 S74 S75 L82 L83 | L84 S76 S77 S78 L85 L86 L87 S79 S80 S81 L88 L89 L90 L91 L92 S82 S83 S84 S85 S86 L93 L94
equation "\"d5\" = a1"
equation "\"d7\" = a1"
equation "\"d9\" = a1"
equation "\"d42\" = a2"
equation "\"d43\" = a2"
equation "\"d44\" = a2"
equation "\"d90\" = a4"
